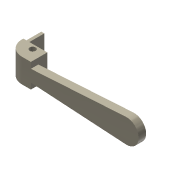
# Autodesk Inventor part: handle
Saved by Autodesk Inventor 2022 Beta2 (Build 260130000, 130) ContinuousBuild 0
## iProperties
Shininess: 64.0
Length Units: 11272
Angle Units: 11279
Time Units: 11290
Mass Units: 11286
Length Display Precision: 3
Angle Display Precision: 2
Created: 2002-01-23
Part Number: handle
Vendor: Unknown
Document SubType Name: Modeling
Designer: Administrator
Density: 1 g/cm^3
Material: Generic
Appearance: Light Beige
Density: 0.0
Volumn: 0.0
Area: 0.0
PropertySet Name: Model Information
Control State: 0
Master: False
Checked Out: False
Author: Administrator
Autodesk Inventor part; units mm, degrees
ref_plane "YZ Plane" through (0, 0, 0) normal (1, 0, 0) x (0, 1, 0)
ref_plane "XZ Plane" through (0, 0, 0) normal (0, 1, 0) x (-1, 0, 0)
ref_plane "XY Plane" through (0, 0, 0) normal (0, 0, 1) x (1, 0, 0)
sketch "Sketch1" plane through (0, 0, 0) normal (0, 0, 1) x (1, 0, 0)
  line L0 (-23.4532, 11.6803) -> (-23.4532, 6.6003)
  line L1 (-23.4532, 6.6003) -> (16.8687, 4.0703)
  arc A0 (16.8687, 4.0703) -> (16.8687, 14.2103) centre (17.1868, 9.1403) ccw
  line L2 (16.8687, 14.2103) -> (-23.4532, 11.6803)
  line L3 (-5.5783, 9.1403) -> (17.1868, 9.1403) construction
  dimension "d0" = 5.08
  dimension "d1" = 40.64
  dimension "d2" = 5.08
  constraints: 8 end point, 2 point on circle, 2 tangent, 1 centre point, 1 coincident, 1 perpendicular, 1 vertical, 1 other
  measures "d0" radius of A0
  measures "d1" horizontal distance of A0.centre L0.end
  measures "d2" distance of L0.start L0.end
extrude "Extrusion1" add sketch "Sketch1" along normal blind 3.175
sketch "Sketch2" plane through (0, 0, 3.175) normal (0, 0, 1) x (1, 0, 0)
  line L0 (-23.4532, 6.6003) -> (-23.4532, 11.6803) projected
  arc A0 (16.8687, 4.0703) -> (16.8687, 14.2103) centre (17.1868, 9.1403) ccw projected
  line L1 (-23.4532, 4.0603) -> (-33.6132, 4.0603)
  line L2 (-33.6132, 4.0603) -> (-33.6132, 14.2203)
  line L3 (-33.6132, 14.2203) -> (-23.4532, 14.2203)
  line L4 (-23.4532, 14.2203) -> (-23.4532, 4.0603)
  line L5 (17.1868, 9.1403) -> (-29.1497, 9.1403) construction
  dimension "d6" = 10.16
  dimension "d7" = 10.16
  dimension "d8" = 5.08
  constraints: 10 end point, 2 horizontal, 2 parallel, 1 collinear, 1 perpendicular
  measures "d6" distance of L2.end L3.end
  measures "d7" distance of L1.end L2.end
  measures "d8" vertical distance of L5.end L1.end
extrude "Extrusion2" add sketch "Sketch2" against normal blind 6.985
sketch "Sketch3" plane through (0, 0, -3.81) normal (0, 0, -1) x (-1, 0, 0)
  line L0 (33.6132, 14.2203) -> (33.6132, 4.0603) projected
  line L1 (32.3432, 12.9503) -> (33.6132, 12.9503)
  line L2 (33.6132, 12.9503) -> (33.6132, 5.3303)
  line L3 (33.6132, 5.3303) -> (32.3432, 5.3303)
  line L4 (32.3432, 5.3303) -> (32.3432, 12.9503)
  dimension "d11" = 1.27
  dimension "d12" = 7.62
  dimension "d13" = 1.27
  constraints: 8 end point, 2 parallel, 1 collinear, 1 horizontal, 1 perpendicular
  measures "d11" distance of L2.end L3.end
  measures "d12" distance of L1.end L2.end
  measures "d13" distance of L0.end L2.end
extrude "Extrusion3" add sketch "Sketch3" along normal blind 7.62
fillet "Fillet1" radius 6.35 1 edges at (-33.6132, 9.1403, 3.175)
sketch "Sketch4" plane through (-33.6132, 14.2203, -3.81) normal (0, 1, 0) x (1, 0, 0)
  point P0 (10.16, 0)
  point P1 (5.842, -1.905)
  dimension "d17" = 4.318
  dimension "d18" = 1.905
  measures "d17" horizontal distance of point (10.16, 0) point (5.842, -1.905)
  measures "d18" vertical distance of point (10.16, 0) point (5.842, -1.905)
hole "Hole1" at (-27.7712, 14.2203, -1.905) direction (0, -1, 0) diameter 2.54 end through all
body "Solid1"
